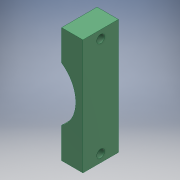
# Autodesk Inventor part: 05-01-Кронштейн низ
Saved by Autodesk Inventor 2018 (Build 220112000, 112)
## iProperties
Part Number: 05-01-Кронштейн низ
Material: Типовые
Document SubType Name: Modeling
Designer: sbnnl
Density: 1 g/cm^3
Appearance: Гладкий — темный цвет морской волны
Author: sbnnl
Autodesk Inventor part; units mm, degrees
ref_plane "YZ Plane" through (0, 0, 0) normal (1, 0, 0) x (0, 1, 0)
ref_plane "XZ Plane" through (0, 0, 0) normal (0, 1, 0) x (-1, 0, 0)
ref_plane "XY Plane" through (0, 0, 0) normal (0, 0, 1) x (1, 0, 0)
sketch "Эскиз1" plane through (0, 0, 0) normal (0, 1, 0) x (-1, 0, 0)
  line L0 (0, 0) -> (12, 0)
  line L1 (12, 0) -> (12, -65) construction
  line L2 (12, -65) -> (0, -65)
  line L3 (0, -65) -> (0, 0)
  line L4 (12, -32.5) -> (76.135, -32.5) construction
  line L5 (4, -10.5388) -> (4, -61.1006) construction
  arc A0 (12, -17.2685) -> (4, -32.5) centre (22.5, -32.5) ccw
  line L6 (12, 0) -> (12, -17.2685)
  line L7 (12, -47.7315) -> (12, -65)
  arc A1 (4, -32.5) -> (12, -47.7315) centre (22.5, -32.5) ccw
  dimension "d0" = 12
  dimension "d1" = 65
  dimension "d3" = 4
  dimension "d4" = 18.5
  constraints: 16 end point, 4 point on circle, 4 point on line, 2 centre point, 2 collinear, 2 horizontal, 2 parallel, 1 midpoint, 1 perpendicular, 1 tangent, 1 vertical
  measures "d0" distance of L1.end L2.end
  measures "d1" distance of L0.end L1.end
  measures "d3" distance between parallel lines of L3 L5
  measures "d4" radius of A0
extrude "Выдавливание1" add sketch "Эскиз1" along normal blind 20
sketch "Эскиз2" plane through (0, 0, 0) normal (1, 0, 0) x (0, 0, -1)
  line L0 (-3.5439, 10) -> (68.6351, 10) construction
  circle A0 centre (4.5, 10) radius 2.25
  circle A1 centre (60.5, 10) radius 2.25
  line L1 (0, 20) -> (65, 20) projected
  line L2 (32.5, 20) -> (32.5, 14.1463) construction
  point P0 (0, 0)
  dimension "d7" = 10
  dimension "d8" = 4.5
  dimension "d9" = 56
  constraints: 4 end point, 2 centre point, 2 point on line, 1 equal radius, 1 horizontal, 1 midpoint, 1 symmetric about line, 1 vertical
  measures "d7" distance from line of L0 point (0, 0)
  measures "d8" diameter of A1
  measures "d9" distance of A1.centre A0.centre
extrude "Выдавливание2" cut sketch "Эскиз2" against normal blind 200
